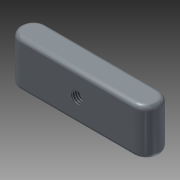
# Autodesk Inventor part: bolt
Saved by Autodesk Inventor 2015 (Build 190159000, 159)
## iProperties
Created: 2015-04-06
Part Number: bolt
Material: Zinc
Document SubType Name: Modeling
Designer: WASHHSST
Density: 7 g/cm^3
Appearance: Zinc
Author: WASHHSST
Autodesk Inventor part; units mm, degrees
ref_plane "YZ Plane" through (0, 0, 0) normal (1, 0, 0) x (0, 1, 0)
ref_plane "XZ Plane" through (0, 0, 0) normal (0, 1, 0) x (-1, 0, 0)
ref_plane "XY Plane" through (0, 0, 0) normal (0, 0, 1) x (1, 0, 0)
sketch "Sketch1" plane through (0, 0, 0) normal (0, 0, 1) x (1, 0, 0)
  line L0 (0, 0) -> (76.2, 0)
  line L1 (76.2, 0) -> (76.2, 25.4)
  line L2 (76.2, 25.4) -> (0, 25.4)
  line L3 (0, 25.4) -> (0, 0)
  dimension "d0" = 76.2
  dimension "d1" = 25.4
  constraints: 8 end point, 2 parallel, 1 horizontal, 1 perpendicular
  measures "d0" distance of L2.end L1.end
  measures "d1" distance of L1.end L0.end
extrude "Extrusion1" add sketch "Sketch1" along normal blind 14.2875
fillet "Fillet1" radius 2.54 8 edges at (38.1, 25.4, 14.2875) (38.1, 0, 14.2875) (76.2, 0, 7.1437) (76.2, 25.4, 7.1437) (0, 25.4, 7.1437) (0, 0, 7.1437) (38.1, 25.4, 0) (38.1, 0, 0)
sketch "Sketch2" plane through (0, 0, 14.2875) normal (0, 0, 1) x (1, 0, 0)
  line L0 (2.54, 2.54) -> (2.54, 22.86) projected
  line L1 (2.54, 12.7) -> (73.66, 12.7)
  line L2 (73.66, 22.86) -> (73.66, 2.54) projected
  circle A0 centre (38.1, 12.7) radius 3.175
  point P0 (0, 0)
  dimension "d5" = 6.35
  constraints: 3 midpoint, 2 end point, 1 centre point
  measures "d5" diameter of A0
extrude "Extrusion2" cut sketch "Sketch2" against normal blind 14.2875
thread "Thread1" size "1/4-20 UNC" class "2B" standard "ANSI Unified Screw Threads" full length
fillet "Fillet2" radius 7.1437 12 edges at (75.4561, 24.6561, 13.5436) (75.4561, 0.7439, 13.5436) (76.2, 12.7, 14.2875) (75.4561, 24.6561, 0.7439) (75.4561, 0.7439, 0.7439) (76.2, 12.7, 0) (0.7439, 0.7439, 13.5436) (0.7439, 24.6561, 13.5436) (0, 12.7, 14.2875) (0.7439, 0.7439, 0.7439) (0.7439, 24.6561, 0.7439) (0, 12.7, 0)
body "Solid1"
